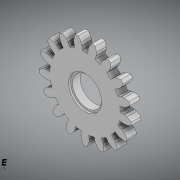
# Autodesk Inventor part: m2z17
Saved by Autodesk Inventor 2020 (Build 240168000, 168)
## iProperties
Created: 2019-12-19
Part Number: m2z17
Material: 一般
Document SubType Name: Modeling
Designer: hamaa
Density: 1 g/cm^3
Appearance: 既定
Author: hamaa
Autodesk Inventor part; units mm, degrees
ref_plane "YZ Plane" through (0, 0, 0) normal (1, 0, 0) x (0, 1, 0)
ref_plane "XZ Plane" through (0, 0, 0) normal (0, 1, 0) x (-1, 0, 0)
ref_plane "XY Plane" through (0, 0, 0) normal (0, 0, 1) x (1, 0, 0)
sketch "スケッチ1" plane through (0, 0, 0) normal (0, 0, 1) x (1, 0, 0)
  arc A0 (149.791, 121.195) -> (149.7368, 120.9269) centre (151.454, 120.7196) ccw
  arc A1 (150.1592, 122.1118) -> (149.791, 121.195) centre (154.3867, 119.8813) ccw
  arc A2 (151.3266, 123.7887) -> (150.1592, 122.1118) centre (157.5466, 118.214) ccw
  arc A3 (143.8535, 120.5678) -> (143.8999, 120.2982) centre (145.576, 120.7252) ccw
  arc A4 (143.8657, 121.5557) -> (143.8535, 120.5678) centre (148.6135, 121.0029) ccw
  arc A5 (144.3485, 123.541) -> (143.8657, 121.5557) centre (152.1623, 120.5898) ccw
  arc A6 (138.5436, 117.838) -> (138.6842, 117.6034) centre (140.0929, 118.6071) ccw
  arc A7 (138.1981, 118.7637) -> (138.5436, 117.838) centre (142.825, 119.9633) ccw
  arc A8 (137.9311, 120.7893) -> (138.1981, 118.7637) centre (146.2834, 120.86) ccw
  arc A9 (134.5784, 113.3745) -> (134.7942, 113.2065) centre (135.7452, 114.6513) ccw
  arc A10 (133.9218, 114.1128) -> (134.5784, 113.3745) centre (137.8029, 116.9028) ccw
  arc A11 (132.941, 115.9052) -> (133.9218, 114.1128) centre (140.7038, 118.9883) ccw
  arc A12 (132.4933, 107.7799) -> (132.7552, 107.7012) centre (133.1201, 109.392) ccw
  arc A13 (131.6144, 108.2312) -> (132.4933, 107.7799) centre (134.2255, 112.2348) ccw
  arc A14 (130.0524, 109.5482) -> (131.6144, 108.2312) centre (136.1771, 115.2274) ccw
  arc A15 (132.57, 101.8099) -> (132.8427, 101.8312) centre (132.5721, 103.5396) ccw
  arc A16 (131.5874, 101.9132) -> (132.57, 101.8099) centre (132.5759, 106.5897) ccw
  arc A17 (129.6551, 102.5771) -> (131.5874, 101.9132) centre (133.3147, 110.0853) ccw
  arc A18 (134.7982, 96.2708) -> (135.0447, 96.3891) centre (134.1753, 97.8844) ccw
  arc A19 (133.8446, 96.0122) -> (134.7982, 96.2708) centre (133.077, 100.73) ccw
  arc A20 (131.803, 95.9331) -> (133.8446, 96.0122) centre (132.5032, 104.2564) ccw
  arc A21 (138.8768, 91.9106) -> (139.064, 92.11) centre (137.7131, 93.1903) ccw
  arc A22 (138.0811, 91.325) -> (138.8768, 91.9106) centre (135.661, 95.4469) ccw
  arc A23 (136.2059, 90.5138) -> (138.0811, 91.325) centre (133.8521, 98.5279) ccw
  arc A24 (144.2552, 89.3182) -> (144.3576, 89.5718) centre (142.7078, 90.0911) ccw
  arc A25 (143.7247, 88.4847) -> (144.2552, 89.3182) centre (139.979, 91.454) ccw
  arc A26 (142.2691, 87.0508) -> (143.7247, 88.4847) centre (137.1793, 93.6735) ccw
  arc A27 (150.2068, 88.8438) -> (150.2107, 89.1172) centre (148.4847, 89.0055) ccw
  arc A28 (150.0132, 87.8749) -> (150.2068, 88.8438) centre (145.4478, 89.2907) ccw
  arc A29 (149.1739, 86.0121) -> (150.0132, 87.8749) centre (142.0354, 90.3489) ccw
  arc A30 (155.9279, 90.5513) -> (155.8328, 90.8078) centre (154.2636, 90.08) ccw
  arc A31 (156.0974, 89.578) -> (155.9279, 90.5513) centre (151.3289, 89.2489) ccw
  arc A32 (155.9877, 87.5378) -> (156.0974, 89.578) centre (147.7646, 89.003) ccw
  arc A33 (160.6458, 94.2103) -> (160.4645, 94.4151) centre (159.2642, 93.1696) ccw
  arc A34 (161.1555, 93.3639) -> (160.6458, 94.2103) centre (156.8278, 91.3345) ccw
  arc A35 (161.7902, 91.4218) -> (161.1555, 93.3639) centre (153.5931, 89.8176) ccw
  arc A36 (163.7233, 99.3265) -> (163.4803, 99.4519) centre (162.811, 97.857) ccw
  arc A37 (164.5044, 98.7214) -> (163.7233, 99.3265) centre (161.2021, 95.2657) ccw
  arc A38 (165.7978, 97.1397) -> (164.5044, 98.7214) centre (158.7337, 92.6826) ccw
  arc A39 (164.7449, 105.2089) -> (164.4729, 105.2381) centre (164.425, 103.5091) ccw
  arc A40 (165.6918, 104.9268) -> (164.7449, 105.2089) centre (163.8608, 100.5115) ccw
  arc A41 (167.4692, 103.9192) -> (165.6918, 104.9268) centre (162.4922, 97.2113) ccw
  arc A42 (163.5725, 111.0631) -> (163.3084, 110.9921) centre (163.8882, 109.3625) ccw
  arc A43 (164.5573, 111.1421) -> (163.5725, 111.0631) centre (164.445, 106.3636) ccw
  arc A44 (166.5787, 110.8447) -> (164.5573, 111.1421) centre (164.361, 102.7918) ccw
  arc A45 (160.3645, 116.0985) -> (160.1438, 115.9369) centre (161.2732, 114.6268) ccw
  arc A46 (161.2543, 116.528) -> (160.3645, 116.0985) centre (162.8757, 112.0315) ccw
  arc A47 (163.2466, 116.9808) -> (161.2543, 116.528) centre (164.0877, 108.6706) ccw
  arc A48 (155.5541, 119.635) -> (155.4067, 119.4046) centre (156.9331, 118.591) ccw
  arc A49 (156.2287, 120.3569) -> (155.5541, 119.635) centre (159.3649, 116.7498) ccw
  arc A50 (157.9229, 121.4989) -> (156.2287, 120.3569) centre (161.7092, 114.0537) ccw
  arc A51 (147.2631, 120.9269) -> (147.209, 121.195) centre (145.5459, 120.7196) ccw
  arc A52 (147.209, 121.195) -> (146.8407, 122.1118) centre (142.6132, 119.8813) ccw
  arc A53 (146.8407, 122.1118) -> (145.6734, 123.7887) centre (139.4533, 118.214) ccw
  arc A54 (141.5932, 119.4046) -> (141.4459, 119.635) centre (140.0669, 118.591) ccw
  arc A55 (141.4459, 119.635) -> (140.7713, 120.3569) centre (137.635, 116.7498) ccw
  arc A56 (140.7713, 120.3569) -> (139.077, 121.4989) centre (135.2908, 114.0537) ccw
  arc A57 (136.8561, 115.9369) -> (136.6355, 116.0985) centre (135.7268, 114.6268) ccw
  arc A58 (136.6355, 116.0985) -> (135.7457, 116.528) centre (134.1242, 112.0315) ccw
  arc A59 (135.7457, 116.528) -> (133.7533, 116.9808) centre (132.9122, 108.6706) ccw
  arc A60 (133.6916, 110.9921) -> (133.4275, 111.0631) centre (133.1117, 109.3625) ccw
  arc A61 (133.4275, 111.0631) -> (132.4426, 111.1421) centre (132.5549, 106.3636) ccw
  arc A62 (132.4426, 111.1421) -> (130.4212, 110.8447) centre (132.6389, 102.7918) ccw
  arc A63 (132.527, 105.2381) -> (132.2551, 105.2089) centre (132.575, 103.5091) ccw
  arc A64 (132.2551, 105.2089) -> (131.3082, 104.9268) centre (133.1391, 100.5115) ccw
  arc A65 (131.3082, 104.9268) -> (129.5307, 103.9192) centre (134.5077, 97.2113) ccw
  arc A66 (133.5197, 99.4519) -> (133.2766, 99.3265) centre (134.189, 97.857) ccw
  arc A67 (133.2766, 99.3265) -> (132.4956, 98.7214) centre (135.7979, 95.2657) ccw
  arc A68 (132.4956, 98.7214) -> (131.2022, 97.1397) centre (138.2662, 92.6826) ccw
  arc A69 (136.5355, 94.4151) -> (136.3542, 94.2103) centre (137.7358, 93.1696) ccw
  arc A70 (136.3542, 94.2103) -> (135.8445, 93.3639) centre (140.1721, 91.3345) ccw
  arc A71 (135.8445, 93.3639) -> (135.2098, 91.4218) centre (143.4069, 89.8176) ccw
  arc A72 (141.1672, 90.8078) -> (141.0721, 90.5513) centre (142.7363, 90.08) ccw
  arc A73 (141.0721, 90.5513) -> (140.9026, 89.578) centre (145.6711, 89.2489) ccw
  arc A74 (140.9026, 89.578) -> (141.0123, 87.5378) centre (149.2354, 89.003) ccw
  arc A75 (146.7892, 89.1172) -> (146.7932, 88.8438) centre (148.5153, 89.0055) ccw
  arc A76 (146.7932, 88.8438) -> (146.9867, 87.8749) centre (151.5521, 89.2907) ccw
  arc A77 (146.9867, 87.8749) -> (147.826, 86.0121) centre (154.9646, 90.3489) ccw
  arc A78 (152.6423, 89.5718) -> (152.7448, 89.3182) centre (154.2922, 90.0911) ccw
  arc A79 (152.7448, 89.3182) -> (153.2753, 88.4847) centre (157.0209, 91.454) ccw
  arc A80 (153.2753, 88.4847) -> (154.7308, 87.0508) centre (159.8207, 93.6735) ccw
  arc A81 (157.9359, 92.11) -> (158.1231, 91.9106) centre (159.2868, 93.1903) ccw
  arc A82 (158.1231, 91.9106) -> (158.9189, 91.325) centre (161.3389, 95.4469) ccw
  arc A83 (158.9189, 91.325) -> (160.7941, 90.5138) centre (163.1478, 98.5279) ccw
  arc A84 (161.9552, 96.3891) -> (162.2018, 96.2708) centre (162.8246, 97.8844) ccw
  arc A85 (162.2018, 96.2708) -> (163.1553, 96.0122) centre (163.923, 100.73) ccw
  arc A86 (163.1553, 96.0122) -> (165.197, 95.9331) centre (164.4967, 104.2564) ccw
  arc A87 (164.1573, 101.8312) -> (164.4299, 101.8099) centre (164.4278, 103.5396) ccw
  arc A88 (164.4299, 101.8099) -> (165.4125, 101.9132) centre (164.424, 106.5897) ccw
  arc A89 (165.4125, 101.9132) -> (167.3448, 102.5771) centre (163.6852, 110.0853) ccw
  arc A90 (164.2447, 107.7012) -> (164.5067, 107.7799) centre (163.8798, 109.392) ccw
  arc A91 (164.5067, 107.7799) -> (165.3856, 108.2312) centre (162.7745, 112.2348) ccw
  arc A92 (165.3856, 108.2312) -> (166.9476, 109.5482) centre (160.8228, 115.2274) ccw
  arc A93 (162.2057, 113.2065) -> (162.4216, 113.3745) centre (161.2547, 114.6513) ccw
  arc A94 (162.4216, 113.3745) -> (163.0781, 114.1128) centre (159.1971, 116.9028) ccw
  arc A95 (163.0781, 114.1128) -> (164.0589, 115.9052) centre (156.2961, 118.9883) ccw
  arc A96 (158.3157, 117.6034) -> (158.4563, 117.838) centre (156.9071, 118.6071) ccw
  arc A97 (158.4563, 117.838) -> (158.8018, 118.7637) centre (154.175, 119.9633) ccw
  arc A98 (158.8018, 118.7637) -> (159.0689, 120.7893) centre (150.7166, 120.86) ccw
  arc A99 (153.1001, 120.2982) -> (153.1464, 120.5678) centre (151.4239, 120.7252) ccw
  arc A100 (153.1464, 120.5678) -> (153.1342, 121.5557) centre (148.3864, 121.0029) ccw
  arc A101 (153.1342, 121.5557) -> (152.6515, 123.541) centre (144.8376, 120.5898) ccw
  arc A102 (149.6227, 119.4566) -> (147.3773, 119.4566) centre (148.5, 105.0001) ccw
  arc A103 (144.3246, 118.8859) -> (142.2308, 118.0748) centre (148.5, 105.0001) ccw
  arc A104 (139.5904, 116.4399) -> (137.931, 114.9272) centre (148.5, 105.0001) ccw
  arc A105 (136.0595, 112.4489) -> (135.0586, 110.4389) centre (148.5, 105.0001) ccw
  arc A106 (134.2088, 107.4519) -> (134.0016, 105.2161) centre (148.5, 105.0001) ccw
  arc A107 (134.2881, 102.1237) -> (134.9026, 99.9641) centre (148.5, 105.0001) ccw
  arc A108 (136.2869, 97.1841) -> (137.64, 95.3922) centre (148.5, 105.0001) ccw
  arc A109 (139.9351, 93.3) -> (141.8441, 92.118) centre (148.5, 105.0001) ccw
  arc A110 (144.74, 90.9961) -> (146.9472, 90.5835) centre (148.5, 105.0001) ccw
  arc A111 (150.0528, 90.5835) -> (152.2599, 90.9961) centre (148.5, 105.0001) ccw
  arc A112 (155.1558, 92.118) -> (157.0648, 93.3) centre (148.5, 105.0001) ccw
  arc A113 (159.3599, 95.3922) -> (160.7131, 97.1841) centre (148.5, 105.0001) ccw
  arc A114 (162.0973, 99.9641) -> (162.7118, 102.1237) centre (148.5, 105.0001) ccw
  arc A115 (162.9984, 105.2161) -> (162.7912, 107.4519) centre (148.5, 105.0001) ccw
  arc A116 (161.9413, 110.4389) -> (160.9405, 112.4489) centre (148.5, 105.0001) ccw
  arc A117 (159.0689, 114.9272) -> (157.4096, 116.4399) centre (148.5, 105.0001) ccw
  arc A118 (154.7691, 118.0748) -> (152.6754, 118.8859) centre (148.5, 105.0001) ccw
  arc A119 (145.6734, 123.7887) -> (144.3485, 123.541) centre (148.5, 105.0001) ccw
  arc A120 (139.077, 121.4989) -> (137.9311, 120.7893) centre (148.5, 105.0001) ccw
  arc A121 (133.7533, 116.9808) -> (132.941, 115.9052) centre (148.5, 105.0001) ccw
  arc A122 (130.4212, 110.8447) -> (130.0524, 109.5482) centre (148.5, 105.0001) ccw
  arc A123 (129.5307, 103.9192) -> (129.6551, 102.5771) centre (148.5, 105.0001) ccw
  arc A124 (131.2022, 97.1397) -> (131.803, 95.9331) centre (148.5, 105.0001) ccw
  arc A125 (135.2098, 91.4218) -> (136.2059, 90.5138) centre (148.5, 105.0001) ccw
  arc A126 (141.0123, 87.5378) -> (142.2691, 87.0508) centre (148.5, 105.0001) ccw
  arc A127 (147.826, 86.0121) -> (149.1739, 86.0121) centre (148.5, 105.0001) ccw
  arc A128 (154.7308, 87.0508) -> (155.9877, 87.5378) centre (148.5, 105.0001) ccw
  arc A129 (160.7941, 90.5138) -> (161.7902, 91.4218) centre (148.5, 105.0001) ccw
  arc A130 (165.197, 95.9331) -> (165.7978, 97.1397) centre (148.5, 105.0001) ccw
  arc A131 (167.3448, 102.5771) -> (167.4692, 103.9192) centre (148.5, 105.0001) ccw
  arc A132 (166.9476, 109.5482) -> (166.5787, 110.8447) centre (148.5, 105.0001) ccw
  arc A133 (164.0589, 115.9052) -> (163.2466, 116.9808) centre (148.5, 105.0001) ccw
  arc A134 (159.0689, 120.7893) -> (157.9229, 121.4989) centre (148.5, 105.0001) ccw
  arc A135 (152.6515, 123.541) -> (151.3266, 123.7887) centre (148.5, 105.0001) ccw
  line L0 (149.6227, 119.4566) -> (149.7368, 120.9269)
  line L1 (144.3246, 118.8859) -> (143.8999, 120.2982)
  line L2 (139.5904, 116.4399) -> (138.6842, 117.6034)
  line L3 (136.0595, 112.4489) -> (134.7942, 113.2065)
  line L4 (134.2088, 107.4519) -> (132.7552, 107.7012)
  line L5 (134.2881, 102.1237) -> (132.8427, 101.8312)
  line L6 (136.2869, 97.1841) -> (135.0447, 96.3891)
  line L7 (139.9351, 93.3) -> (139.064, 92.11)
  line L8 (144.74, 90.9961) -> (144.3576, 89.5718)
  line L9 (150.0528, 90.5835) -> (150.2107, 89.1172)
  line L10 (155.1558, 92.118) -> (155.8328, 90.8078)
  line L11 (159.3599, 95.3922) -> (160.4645, 94.4151)
  line L12 (162.0973, 99.9641) -> (163.4803, 99.4519)
  line L13 (162.9984, 105.2161) -> (164.4729, 105.2381)
  line L14 (161.9413, 110.4389) -> (163.3084, 110.9921)
  line L15 (159.0689, 114.9272) -> (160.1438, 115.9369)
  line L16 (154.7691, 118.0748) -> (155.4067, 119.4046)
  line L17 (147.3773, 119.4566) -> (147.2631, 120.9269)
  line L18 (142.2308, 118.0748) -> (141.5932, 119.4046)
  line L19 (137.931, 114.9272) -> (136.8561, 115.9369)
  line L20 (135.0586, 110.4389) -> (133.6916, 110.9921)
  line L21 (134.0016, 105.2161) -> (132.527, 105.2381)
  line L22 (134.9026, 99.9641) -> (133.5197, 99.4519)
  line L23 (137.64, 95.3922) -> (136.5355, 94.4151)
  line L24 (141.8441, 92.118) -> (141.1672, 90.8078)
  line L25 (146.9472, 90.5835) -> (146.7892, 89.1172)
  line L26 (152.2599, 90.9961) -> (152.6423, 89.5718)
  line L27 (157.0648, 93.3) -> (157.9359, 92.11)
  line L28 (160.7131, 97.1841) -> (161.9552, 96.3891)
  line L29 (162.7118, 102.1237) -> (164.1573, 101.8312)
  line L30 (162.7912, 107.4519) -> (164.2447, 107.7012)
  line L31 (160.9405, 112.4489) -> (162.2057, 113.2065)
  line L32 (157.4096, 116.4399) -> (158.3157, 117.6034)
  line L33 (152.6754, 118.8859) -> (153.1001, 120.2982)
  line L34 (127.5, 105) -> (169.5, 105)
  line L35 (148.5, 84) -> (148.5, 126)
  line L36 (187.5, 124.0001) -> (257.5, 124.0001)
  line L37 (187.5, 116.0001) -> (257.5, 116.0001)
  line L38 (187.5, 108.0001) -> (257.5, 108.0001)
  line L39 (187.5, 100.0001) -> (257.5, 100.0001)
  line L40 (187.5, 92.0001) -> (257.5, 92.0001)
  line L41 (187.5, 84.0001) -> (257.5, 84.0001)
  line L42 (187.5, 76.0001) -> (257.5, 76.0001)
  line L43 (187.5, 68.0001) -> (257.5, 68.0001)
  line L44 (187.5, 60.0001) -> (257.5, 60.0001)
  line L45 (187.5, 52.0001) -> (257.5, 52.0001)
  line L46 (187.5, 44.0001) -> (257.5, 44.0001)
  line L47 (187.5, 36.0001) -> (257.5, 36.0001)
  line L48 (187.5, 28.0001) -> (257.5, 28.0001)
  line L49 (187.5, 124.0001) -> (187.5, 28.0001)
  line L50 (257.5, 124.0001) -> (257.5, 28.0001)
  line L51 (222.5, 116.0001) -> (222.5, 28.0001)
  point P0 (0, 0)
  point P1 (193.5, 118)
  point P2 (196, 110)
  point P3 (196, 102)
  point P4 (193.5, 94)
  point P5 (196, 86)
  point P6 (191, 78)
  point P7 (193.5, 70)
  point P8 (193.5, 62)
  point P9 (193.5, 54)
  point P10 (196, 46)
  point P11 (196, 38)
  point P12 (193.5, 30)
  point P13 (223.5, 110)
  point P14 (238.5, 102)
  point P15 (239.75, 94)
  point P16 (236, 86)
  point P17 (238.5, 78)
  point P18 (232.25, 70)
  point P19 (238.5, 62)
  point P20 (238.5, 54)
  point P21 (233.5, 46)
  point P22 (241, 38)
  point P23 (241, 30)
  point P24 (149.5, 139.5)
  point P25 (149.5, 133.5)
  point P26 (166.75, 139.5)
  point P27 (167.8125, 133.5)
  constraints: 204 point on circle, 102 centre point, 100 end point, 99 equal radius, 68 tangent, 19 horizontal, 13 parallel, 2 horizontal alignment, 2 midpoint, 2 perpendicular, 155 other
extrude "押し出し1" add sketch "スケッチ1" along normal blind 4 contours A1 A2 A135 A101 A100 A99 L33 A118 L16 A48 A49 A50 A134 A98 A97 A96 L32 A117 L15 A45 A46 A47 A133 A95 A94 A93 L31 A116 L14 A42 A43 A44 A132 A92 A91 A90 L30 A115 L13 A39 A40 L34 L35 A102 L0 A0 | L35 L34 A64 A63 L21 A106 L4 A12 A13 A14 A122 A62 A61 A60 L20 A105 L3 A9 A10 A11 A121 A59 A58 A57 L19 A104 L2 A6 A7 A8 A120 A56 A55 A54 L18 A103 L1 A3 A4 A5 A119 A53 A52 A51 L17 A102 | L35 A127 A77 A76 A75 L25 A110 L8 A24 A25 A26 A126 A74 A73 A72 L24 A109 L7 A21 A22 A23 A125 A71 A70 A69 L23 A108 L6 A18 A19 A20 A124 A68 A67 A66 L22 A107 L5 A15 A16 A17 A123 A65 A64 L34 | L34 A40 A41 A131 A89 A88 A87 L29 A114 L12 A36 A37 A38 A130 A86 A85 A84 L28 A113 L11 A33 A34 A35 A129 A83 A82 A81 L27 A112 L10 A30 A31 A32 A128 A80 A79 A78 L26 A111 L9 A27 A28 A29 A127 L35
sketch "スケッチ2" plane through (0, 0, 4) normal (0, 0, 1) x (1, 0, 0)
  line L0 (137.931, 114.9272) -> (136.8561, 115.9369) projected
  arc A0 (136.8561, 115.9369) -> (136.6355, 116.0985) centre (135.7268, 114.6268) ccw projected
  arc A1 (136.6355, 116.0985) -> (135.7457, 116.528) centre (134.1242, 112.0315) ccw projected
  arc A2 (135.7457, 116.528) -> (133.7533, 116.9808) centre (132.9122, 108.6706) ccw projected
  arc A3 (133.7533, 116.9808) -> (132.941, 115.9052) centre (148.5, 105.0001) ccw projected
  arc A4 (132.941, 115.9052) -> (133.9218, 114.1128) centre (140.7038, 118.9883) ccw projected
  arc A5 (133.9218, 114.1128) -> (134.5784, 113.3745) centre (137.8029, 116.9028) ccw projected
  arc A6 (134.5784, 113.3745) -> (134.7942, 113.2065) centre (135.7452, 114.6513) ccw projected
  line L1 (134.7942, 113.2065) -> (136.0595, 112.4489) projected
  arc A7 (136.0595, 112.4489) -> (135.0586, 110.4389) centre (148.5, 105.0001) ccw projected
  line L2 (135.0586, 110.4389) -> (133.6916, 110.9921) projected
  arc A8 (133.6916, 110.9921) -> (133.4275, 111.0631) centre (133.1117, 109.3625) ccw projected
  arc A9 (133.4275, 111.0631) -> (132.4426, 111.1421) centre (132.5549, 106.3636) ccw projected
  arc A10 (132.4426, 111.1421) -> (130.4212, 110.8447) centre (132.6389, 102.7918) ccw projected
  arc A11 (130.4212, 110.8447) -> (130.0524, 109.5482) centre (148.5, 105.0001) ccw projected
  arc A12 (130.0524, 109.5482) -> (131.6144, 108.2312) centre (136.1771, 115.2274) ccw projected
  arc A13 (131.6144, 108.2312) -> (132.4933, 107.7799) centre (134.2255, 112.2348) ccw projected
  arc A14 (132.4933, 107.7799) -> (132.7552, 107.7012) centre (133.1201, 109.392) ccw projected
  line L3 (132.7552, 107.7012) -> (134.2088, 107.4519) projected
  arc A15 (134.2088, 107.4519) -> (134.0016, 105.2161) centre (148.5, 105.0001) ccw projected
  line L4 (134.0016, 105.2161) -> (132.527, 105.2381) projected
  arc A16 (132.527, 105.2381) -> (132.2551, 105.2089) centre (132.575, 103.5091) ccw projected
  arc A17 (132.2551, 105.2089) -> (131.3082, 104.9268) centre (133.1391, 100.5115) ccw projected
  arc A18 (131.3082, 104.9268) -> (129.5307, 103.9192) centre (134.5077, 97.2113) ccw projected
  arc A19 (129.5307, 103.9192) -> (129.6551, 102.5771) centre (148.5, 105.0001) ccw projected
  arc A20 (129.6551, 102.5771) -> (131.5874, 101.9132) centre (133.3147, 110.0853) ccw projected
  arc A21 (131.5874, 101.9132) -> (132.57, 101.8099) centre (132.5759, 106.5897) ccw projected
  arc A22 (132.57, 101.8099) -> (132.8427, 101.8312) centre (132.5721, 103.5396) ccw projected
  line L5 (132.8427, 101.8312) -> (134.2881, 102.1237) projected
  arc A23 (134.2881, 102.1237) -> (134.9026, 99.9641) centre (148.5, 105.0001) ccw projected
  line L6 (134.9026, 99.9641) -> (133.5197, 99.4519) projected
  arc A24 (133.5197, 99.4519) -> (133.2766, 99.3265) centre (134.189, 97.857) ccw projected
  arc A25 (133.2766, 99.3265) -> (132.4956, 98.7214) centre (135.7979, 95.2657) ccw projected
  arc A26 (132.4956, 98.7214) -> (131.2022, 97.1397) centre (138.2662, 92.6826) ccw projected
  arc A27 (131.2022, 97.1397) -> (131.803, 95.9331) centre (148.5, 105.0001) ccw projected
  arc A28 (131.803, 95.9331) -> (133.8446, 96.0122) centre (132.5032, 104.2564) ccw projected
  arc A29 (133.8446, 96.0122) -> (134.7982, 96.2708) centre (133.077, 100.73) ccw projected
  arc A30 (134.7982, 96.2708) -> (135.0447, 96.3891) centre (134.1753, 97.8844) ccw projected
  line L7 (135.0447, 96.3891) -> (136.2869, 97.1841) projected
  arc A31 (136.2869, 97.1841) -> (137.64, 95.3922) centre (148.5, 105.0001) ccw projected
  line L8 (137.64, 95.3922) -> (136.5355, 94.4151) projected
  arc A32 (136.5355, 94.4151) -> (136.3542, 94.2103) centre (137.7358, 93.1696) ccw projected
  arc A33 (136.3542, 94.2103) -> (135.8445, 93.3639) centre (140.1721, 91.3345) ccw projected
  arc A34 (135.8445, 93.3639) -> (135.2098, 91.4218) centre (143.4069, 89.8176) ccw projected
  arc A35 (135.2098, 91.4218) -> (136.2059, 90.5138) centre (148.5, 105.0001) ccw projected
  arc A36 (136.2059, 90.5138) -> (138.0811, 91.325) centre (133.8521, 98.5279) ccw projected
  arc A37 (138.0811, 91.325) -> (138.8768, 91.9106) centre (135.661, 95.4469) ccw projected
  arc A38 (138.8768, 91.9106) -> (139.064, 92.11) centre (137.7131, 93.1903) ccw projected
  line L9 (139.064, 92.11) -> (139.9351, 93.3) projected
  arc A39 (139.9351, 93.3) -> (141.8441, 92.118) centre (148.5, 105.0001) ccw projected
  line L10 (141.8441, 92.118) -> (141.1672, 90.8078) projected
  arc A40 (141.1672, 90.8078) -> (141.0721, 90.5513) centre (142.7363, 90.08) ccw projected
  arc A41 (141.0721, 90.5513) -> (140.9026, 89.578) centre (145.6711, 89.2489) ccw projected
  arc A42 (140.9026, 89.578) -> (141.0123, 87.5378) centre (149.2354, 89.003) ccw projected
  arc A43 (141.0123, 87.5378) -> (142.2691, 87.0508) centre (148.5, 105.0001) ccw projected
  arc A44 (142.2691, 87.0508) -> (143.7247, 88.4847) centre (137.1793, 93.6735) ccw projected
  arc A45 (143.7247, 88.4847) -> (144.2552, 89.3182) centre (139.979, 91.454) ccw projected
  arc A46 (144.2552, 89.3182) -> (144.3576, 89.5718) centre (142.7078, 90.0911) ccw projected
  line L11 (144.3576, 89.5718) -> (144.74, 90.9961) projected
  arc A47 (144.74, 90.9961) -> (146.9472, 90.5835) centre (148.5, 105.0001) ccw projected
  line L12 (146.9472, 90.5835) -> (146.7892, 89.1172) projected
  arc A48 (146.7892, 89.1172) -> (146.7932, 88.8438) centre (148.5153, 89.0055) ccw projected
  arc A49 (146.7932, 88.8438) -> (146.9867, 87.8749) centre (151.5521, 89.2907) ccw projected
  arc A50 (146.9867, 87.8749) -> (147.826, 86.0121) centre (154.9646, 90.3489) ccw projected
  arc A51 (147.826, 86.0121) -> (149.1739, 86.0121) centre (148.5, 105.0001) ccw projected
  arc A52 (149.1739, 86.0121) -> (150.0132, 87.8749) centre (142.0354, 90.3489) ccw projected
  arc A53 (150.0132, 87.8749) -> (150.2068, 88.8438) centre (145.4478, 89.2907) ccw projected
  arc A54 (150.2068, 88.8438) -> (150.2107, 89.1172) centre (148.4847, 89.0055) ccw projected
  line L13 (150.2107, 89.1172) -> (150.0528, 90.5835) projected
  arc A55 (150.0528, 90.5835) -> (152.2599, 90.9961) centre (148.5, 105.0001) ccw projected
  line L14 (152.2599, 90.9961) -> (152.6423, 89.5718) projected
  arc A56 (152.6423, 89.5718) -> (152.7448, 89.3182) centre (154.2922, 90.0911) ccw projected
  arc A57 (152.7448, 89.3182) -> (153.2753, 88.4847) centre (157.0209, 91.454) ccw projected
  arc A58 (153.2753, 88.4847) -> (154.7308, 87.0508) centre (159.8207, 93.6735) ccw projected
  arc A59 (154.7308, 87.0508) -> (155.9877, 87.5378) centre (148.5, 105.0001) ccw projected
  arc A60 (155.9877, 87.5378) -> (156.0974, 89.578) centre (147.7646, 89.003) ccw projected
  arc A61 (156.0974, 89.578) -> (155.9279, 90.5513) centre (151.3289, 89.2489) ccw projected
  arc A62 (155.9279, 90.5513) -> (155.8328, 90.8078) centre (154.2636, 90.08) ccw projected
  line L15 (155.8328, 90.8078) -> (155.1558, 92.118) projected
  arc A63 (155.1558, 92.118) -> (157.0648, 93.3) centre (148.5, 105.0001) ccw projected
  line L16 (157.0648, 93.3) -> (157.9359, 92.11) projected
  arc A64 (157.9359, 92.11) -> (158.1231, 91.9106) centre (159.2868, 93.1903) ccw projected
  arc A65 (158.1231, 91.9106) -> (158.9189, 91.325) centre (161.3389, 95.4469) ccw projected
  arc A66 (158.9189, 91.325) -> (160.7941, 90.5138) centre (163.1478, 98.5279) ccw projected
  arc A67 (160.7941, 90.5138) -> (161.7902, 91.4218) centre (148.5, 105.0001) ccw projected
  arc A68 (161.7902, 91.4218) -> (161.1555, 93.3639) centre (153.5931, 89.8176) ccw projected
  arc A69 (161.1555, 93.3639) -> (160.6458, 94.2103) centre (156.8278, 91.3345) ccw projected
  arc A70 (160.6458, 94.2103) -> (160.4645, 94.4151) centre (159.2642, 93.1696) ccw projected
  line L17 (160.4645, 94.4151) -> (159.3599, 95.3922) projected
  arc A71 (159.3599, 95.3922) -> (160.7131, 97.1841) centre (148.5, 105.0001) ccw projected
  line L18 (160.7131, 97.1841) -> (161.9552, 96.3891) projected
  arc A72 (161.9552, 96.3891) -> (162.2018, 96.2708) centre (162.8246, 97.8844) ccw projected
  arc A73 (162.2018, 96.2708) -> (163.1553, 96.0122) centre (163.923, 100.73) ccw projected
  arc A74 (163.1553, 96.0122) -> (165.197, 95.9331) centre (164.4967, 104.2564) ccw projected
  arc A75 (165.197, 95.9331) -> (165.7978, 97.1397) centre (148.5, 105.0001) ccw projected
  arc A76 (165.7978, 97.1397) -> (164.5044, 98.7214) centre (158.7337, 92.6826) ccw projected
  arc A77 (164.5044, 98.7214) -> (163.7233, 99.3265) centre (161.2021, 95.2657) ccw projected
  arc A78 (163.7233, 99.3265) -> (163.4803, 99.4519) centre (162.811, 97.857) ccw projected
  line L19 (163.4803, 99.4519) -> (162.0973, 99.9641) projected
  arc A79 (162.0973, 99.9641) -> (162.7118, 102.1237) centre (148.5, 105.0001) ccw projected
  line L20 (162.7118, 102.1237) -> (164.1573, 101.8312) projected
  arc A80 (164.1573, 101.8312) -> (164.4299, 101.8099) centre (164.4278, 103.5396) ccw projected
  arc A81 (164.4299, 101.8099) -> (165.4125, 101.9132) centre (164.424, 106.5897) ccw projected
  arc A82 (165.4125, 101.9132) -> (167.3448, 102.5771) centre (163.6852, 110.0853) ccw projected
  arc A83 (167.3448, 102.5771) -> (167.4692, 103.9192) centre (148.5, 105.0001) ccw projected
  arc A84 (167.4692, 103.9192) -> (165.6918, 104.9268) centre (162.4922, 97.2113) ccw projected
  arc A85 (165.6918, 104.9268) -> (164.7449, 105.2089) centre (163.8608, 100.5115) ccw projected
  arc A86 (164.7449, 105.2089) -> (164.4729, 105.2381) centre (164.425, 103.5091) ccw projected
  line L21 (164.4729, 105.2381) -> (162.9984, 105.2161) projected
  arc A87 (162.9984, 105.2161) -> (162.7912, 107.4519) centre (148.5, 105.0001) ccw projected
  line L22 (162.7912, 107.4519) -> (164.2447, 107.7012) projected
  arc A88 (164.2447, 107.7012) -> (164.5067, 107.7799) centre (163.8798, 109.392) ccw projected
  arc A89 (164.5067, 107.7799) -> (165.3856, 108.2312) centre (162.7745, 112.2348) ccw projected
  arc A90 (165.3856, 108.2312) -> (166.9476, 109.5482) centre (160.8228, 115.2274) ccw projected
  arc A91 (166.9476, 109.5482) -> (166.5787, 110.8447) centre (148.5, 105.0001) ccw projected
  arc A92 (166.5787, 110.8447) -> (164.5573, 111.1421) centre (164.361, 102.7918) ccw projected
  arc A93 (164.5573, 111.1421) -> (163.5725, 111.0631) centre (164.445, 106.3636) ccw projected
  arc A94 (163.5725, 111.0631) -> (163.3084, 110.9921) centre (163.8882, 109.3625) ccw projected
  line L23 (163.3084, 110.9921) -> (161.9413, 110.4389) projected
  arc A95 (161.9413, 110.4389) -> (160.9405, 112.4489) centre (148.5, 105.0001) ccw projected
  line L24 (160.9405, 112.4489) -> (162.2057, 113.2065) projected
  arc A96 (162.2057, 113.2065) -> (162.4216, 113.3745) centre (161.2547, 114.6513) ccw projected
  arc A97 (162.4216, 113.3745) -> (163.0781, 114.1128) centre (159.1971, 116.9028) ccw projected
  arc A98 (163.0781, 114.1128) -> (164.0589, 115.9052) centre (156.2961, 118.9883) ccw projected
  arc A99 (164.0589, 115.9052) -> (163.2466, 116.9808) centre (148.5, 105.0001) ccw projected
  arc A100 (163.2466, 116.9808) -> (161.2543, 116.528) centre (164.0877, 108.6706) ccw projected
  arc A101 (161.2543, 116.528) -> (160.3645, 116.0985) centre (162.8757, 112.0315) ccw projected
  arc A102 (160.3645, 116.0985) -> (160.1438, 115.9369) centre (161.2732, 114.6268) ccw projected
  line L25 (160.1438, 115.9369) -> (159.0689, 114.9272) projected
  arc A103 (159.0689, 114.9272) -> (157.4096, 116.4399) centre (148.5, 105.0001) ccw projected
  line L26 (157.4096, 116.4399) -> (158.3157, 117.6034) projected
  arc A104 (158.3157, 117.6034) -> (158.4563, 117.838) centre (156.9071, 118.6071) ccw projected
  arc A105 (158.4563, 117.838) -> (158.8018, 118.7637) centre (154.175, 119.9633) ccw projected
  arc A106 (158.8018, 118.7637) -> (159.0689, 120.7893) centre (150.7166, 120.86) ccw projected
  arc A107 (159.0689, 120.7893) -> (157.9229, 121.4989) centre (148.5, 105.0001) ccw projected
  arc A108 (157.9229, 121.4989) -> (156.2287, 120.3569) centre (161.7092, 114.0537) ccw projected
  arc A109 (156.2287, 120.3569) -> (155.5541, 119.635) centre (159.3649, 116.7498) ccw projected
  arc A110 (155.5541, 119.635) -> (155.4067, 119.4046) centre (156.9331, 118.591) ccw projected
  line L27 (155.4067, 119.4046) -> (154.7691, 118.0748) projected
  arc A111 (154.7691, 118.0748) -> (152.6754, 118.8859) centre (148.5, 105.0001) ccw projected
  line L28 (152.6754, 118.8859) -> (153.1001, 120.2982) projected
  arc A112 (153.1001, 120.2982) -> (153.1464, 120.5678) centre (151.4239, 120.7252) ccw projected
  arc A113 (153.1464, 120.5678) -> (153.1342, 121.5557) centre (148.3864, 121.0029) ccw projected
  arc A114 (153.1342, 121.5557) -> (152.6515, 123.541) centre (144.8376, 120.5898) ccw projected
  arc A115 (152.6515, 123.541) -> (151.3266, 123.7887) centre (148.5, 105.0001) ccw projected
  arc A116 (151.3266, 123.7887) -> (150.1592, 122.1118) centre (157.5466, 118.214) ccw projected
  arc A117 (150.1592, 122.1118) -> (149.791, 121.195) centre (154.3867, 119.8813) ccw projected
  arc A118 (149.791, 121.195) -> (149.7368, 120.9269) centre (151.454, 120.7196) ccw projected
  line L29 (149.7368, 120.9269) -> (149.6227, 119.4566) projected
  arc A119 (149.6227, 119.4566) -> (147.3773, 119.4566) centre (148.5, 105.0001) ccw projected
  line L30 (147.3773, 119.4566) -> (147.2631, 120.9269) projected
  arc A120 (147.2631, 120.9269) -> (147.209, 121.195) centre (145.5459, 120.7196) ccw projected
  arc A121 (147.209, 121.195) -> (146.8407, 122.1118) centre (142.6132, 119.8813) ccw projected
  arc A122 (146.8407, 122.1118) -> (145.6734, 123.7887) centre (139.4533, 118.214) ccw projected
  arc A123 (145.6734, 123.7887) -> (144.3485, 123.541) centre (148.5, 105.0001) ccw projected
  arc A124 (144.3485, 123.541) -> (143.8657, 121.5557) centre (152.1623, 120.5898) ccw projected
  arc A125 (143.8657, 121.5557) -> (143.8535, 120.5678) centre (148.6135, 121.0029) ccw projected
  arc A126 (143.8535, 120.5678) -> (143.8999, 120.2982) centre (145.576, 120.7252) ccw projected
  line L31 (143.8999, 120.2982) -> (144.3246, 118.8859) projected
  arc A127 (144.3246, 118.8859) -> (142.2308, 118.0748) centre (148.5, 105.0001) ccw projected
  line L32 (142.2308, 118.0748) -> (141.5932, 119.4046) projected
  arc A128 (141.5932, 119.4046) -> (141.4459, 119.635) centre (140.0669, 118.591) ccw projected
  arc A129 (141.4459, 119.635) -> (140.7713, 120.3569) centre (137.635, 116.7498) ccw projected
  arc A130 (140.7713, 120.3569) -> (139.077, 121.4989) centre (135.2908, 114.0537) ccw projected
  arc A131 (139.077, 121.4989) -> (137.9311, 120.7893) centre (148.5, 105.0001) ccw projected
  arc A132 (137.9311, 120.7893) -> (138.1981, 118.7637) centre (146.2834, 120.86) ccw projected
  arc A133 (138.1981, 118.7637) -> (138.5436, 117.838) centre (142.825, 119.9633) ccw projected
  arc A134 (138.5436, 117.838) -> (138.6842, 117.6034) centre (140.0929, 118.6071) ccw projected
  line L33 (138.6842, 117.6034) -> (139.5904, 116.4399) projected
  arc A135 (139.5904, 116.4399) -> (137.931, 114.9272) centre (148.5, 105.0001) ccw projected
  circle A136 centre (148.5, 105.0001) radius 6
  circle A137 centre (148.5, 105.0001) radius 6.8
  point P0 (0, 0)
  dimension "d2" = 12
  dimension "d3" = 0.8
  constraints: 2 centre point, 1 coincident
  measures "d2" diameter of A136
  measures "d3" radial gap between concentric circles of A136 A137
extrude "押し出し2" cut sketch "スケッチ2" against normal blind 4 contours A136
extrude "押し出し3" cut sketch "スケッチ2" against normal blind 0.8 contours A136 | A137
